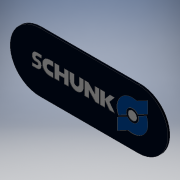
# Autodesk Inventor part: SCHUNK-9905502 Typenschild 9x24x0.3
Saved by Autodesk Inventor 2019 (Build 230136000, 136)
## iProperties
Created: 2022-08-29
Part Number: SCHUNK-9905502 Typenschild 9x24x0.3
Material: Generic
Catalog Web Link: www.cadenas.de
Description: Typenschild-SCHUNK-Typenschild
Vendor: SCHUNK
Document SubType Name: Modeling
Designer: psAdmin
Manufacturer: SCHUNK
Mass: 0.0577878 g
Surface Area: 4.19568 cm^2
Volume: 0.0577878 cm^3
Density: 1 g/cm^3
Appearance: PSOLRGB-175-175-175
Category: PARTsolutions
Company: SCHUNK
Title: SCHUNK-9905502 Typenschild 9x24x0.3
Author: Cadenas PARTsolutions
Comments: SCHUNK-Typenschild
PSOL_IDENT_0: {$CADENAS_DATA/23d-libs/schunk/normteile/typenschilder.prj},215 {VTYP=3D},{NB=SCHUNK-9905502 Typensc
PSOL_IDENT_1: hild 9x24x0.3},{LINA=SCHUNK-9905502 Typenschild 9x24x0.3},{NN=Typenschild},{DATE=31.03.2022 08:21:34
PSOL_IDENT_2: },{GEOMDATE=22.02.2022 09:18:32},{VERSION=},{LINEID=40},{WBVAR=},{WBNUMERIC=}  {NB=SCHUNK-9905502 Ty
PSOL_IDENT_3: penschild 9x24x0.3},{LINA=SCHUNK-9905502 Typenschild 9x24x0.3},{KT=DUMMY},{IDNR=9905502},{TYP=9x24x0
PSOL_IDENT_4: .3},{B=9.000},{L=24.000},{H=0.300},{SF=3.000},{SFL=2.800},{SFS=0.185},{SFBS=2.350},{VBS=-0.320},{VBC=
PSOL_IDENT_5: -0.400},{VBU=0.410},{VL=6.600},{VS=-36.900},{TYP1=4.000},{PARTSERVER=1.000}
NB: SCHUNK-9905502 Typenschild 9x24x0.3
NN: Typenschild
NT: SCHUNK-Typenschild
NBSYN: SCHUNK-$IDNR. Typenschild $TYP.
LINA: SCHUNK-9905502 Typenschild 9x24x0.3
CATALOG: SCHUNK
IDNR: 9905502
TYP: 9x24x0.3
B: 9
L: 24
H: 0.3
SF: 3
SFL: 2.8
SFS: 0.185
SFBS: 2.35
VBS: -0.32
VBC: -0.4
VBU: 0.41
VL: 6.6
VS: -36.9
TYP1: 4
PARTSERVER: 1
SUPPLIER: SCHUNK
ARTICLENO: SCHUNK-9905502 Typenschild 9x24x0.3
BOMINFO: SCHUNK-9905502 Typenschild 9x24x0.3
CREATOR: CADENAS GmbH
Autodesk Inventor part; units mm, degrees
sketch "Sketch_1" plane through (0, 0, 0) normal (0, 0, 1) x (1, 0, 0)
  arc A0 (-12, 0) -> (-7.5, -4.5) centre (-7.5, 0) ccw
  line L0 (-7.5, -4.5) -> (7.5, -4.5)
  arc A1 (7.5, -4.5) -> (12, 0) centre (7.5, 0) ccw
  arc A2 (12, 0) -> (7.5, 4.5) centre (7.5, 0) ccw
  line L1 (7.5, 4.5) -> (-7.5, 4.5)
  arc A3 (-7.5, 4.5) -> (-12, 0) centre (-7.5, 0) ccw
  constraints: 8 point on circle, 4 centre point, 4 end point
extrude "Extrusion1" add sketch "Sketch_1" along normal blind 0.3
sketch "Sketch_13" plane through (0, 0, 0.3) normal (0, 0, 1) x (1, 0, 0)
  line L0 (-5.2261, 1.0265) -> (-5.2261, -1.027)
  line L1 (-5.2261, -1.027) -> (-4.5423, -1.027)
  line L2 (-4.5423, -1.027) -> (-4.5423, -0.2502)
  line L3 (-4.5423, -0.2502) -> (-3.7899, -0.2502)
  line L4 (-3.7899, -0.2502) -> (-3.7899, -1.027)
  line L5 (-3.7899, -1.027) -> (-3.106, -1.027)
  line L6 (-3.106, -1.027) -> (-3.106, 1.0265)
  line L7 (-3.106, 1.0265) -> (-3.7899, 1.0265)
  line L8 (-3.7899, 1.0265) -> (-3.7899, 0.2798)
  line L9 (-3.7899, 0.2798) -> (-4.5423, 0.2798)
  line L10 (-4.5423, 0.2798) -> (-4.5423, 1.0265)
  line L11 (-4.5423, 1.0265) -> (-5.2261, 1.0265)
  constraints: 24 end point
extrude "Extrusion2" cut sketch "Sketch_13" against normal blind 0.05
sketch "Sketch_15" plane through (0, 0, 0.3) normal (0, 0, 1) x (1, 0, 0)
  line L0 (-0.689, 1.0265) -> (-0.689, -1.027)
  line L1 (-0.689, -1.027) -> (-0.0337, -1.027)
  line L2 (-0.0337, -1.027) -> (-0.0337, 0.0269)
  line L3 (-0.0337, 0.0269) -> (0.9535, -1.027)
  line L4 (0.9535, -1.027) -> (1.537, -1.027)
  line L5 (1.537, -1.027) -> (1.537, 1.0265)
  line L6 (1.537, 1.0265) -> (0.8819, 1.0265)
  line L7 (0.8819, 1.0265) -> (0.8819, -0.0273)
  line L8 (0.8819, -0.0273) -> (-0.1051, 1.0265)
  line L9 (-0.1051, 1.0265) -> (-0.689, 1.0265)
  constraints: 20 end point
extrude "Extrusion3" cut sketch "Sketch_15" against normal blind 0.05
sketch "Sketch_16" plane through (0, 0, 0.3) normal (0, 0, 1) x (1, 0, 0)
  line L0 (1.7129, 1.0265) -> (1.7129, -1.027)
  line L1 (1.7129, -1.027) -> (2.3967, -1.027)
  line L2 (2.3967, -1.027) -> (2.3967, -0.0588)
  line L3 (2.3967, -0.0588) -> (3.1093, -1.027)
  line L4 (3.1093, -1.027) -> (3.9246, -1.027)
  line L5 (3.9246, -1.027) -> (3.1004, 0.0719)
  line L6 (3.1004, 0.0719) -> (3.8959, 1.0265)
  line L7 (3.8959, 1.0265) -> (3.1777, 1.0265)
  line L8 (3.1777, 1.0265) -> (2.3967, 0.0961)
  line L9 (2.3967, 0.0961) -> (2.3967, 1.0265)
  line L10 (2.3967, 1.0265) -> (1.7129, 1.0265)
  constraints: 22 end point
extrude "Extrusion4" cut sketch "Sketch_16" against normal blind 0.05
sketch "Sketch_5" plane through (0, 0, 0.3) normal (0, 0, 1) x (1, 0, 0)
  arc A0 (-8.6625, 0.2585) -> (-8.1925, -0.2115) centre (-8.1925, 0.2585) ccw
  line L0 (-8.1925, -0.2115) -> (-7.9457, -0.2115)
  arc A1 (-7.9457, -0.611) -> (-7.9457, -0.2115) centre (-7.9457, -0.4113) ccw
  line L1 (-7.9457, -0.611) -> (-8.6625, -0.611)
  line L2 (-8.6625, -0.611) -> (-8.6625, -1.0575)
  line L3 (-8.6625, -1.0575) -> (-7.9105, -1.0575)
  arc A2 (-7.9105, -1.0575) -> (-7.2525, -0.3995) centre (-7.9105, -0.3995) ccw
  line L4 (-7.2525, -0.3995) -> (-7.2525, -0.2585)
  arc A3 (-7.2525, -0.2585) -> (-7.7225, 0.2115) centre (-7.7225, -0.2585) ccw
  line L5 (-7.7225, 0.2115) -> (-7.9457, 0.2115)
  arc A4 (-7.9457, 0.611) -> (-7.9457, 0.2115) centre (-7.9395, 0.4113) ccw
  line L6 (-7.9457, 0.611) -> (-7.2525, 0.611)
  line L7 (-7.2525, 0.611) -> (-7.2525, 1.0575)
  line L8 (-7.2525, 1.0575) -> (-8.0045, 1.0575)
  arc A5 (-8.0045, 1.0575) -> (-8.6625, 0.3995) centre (-8.0045, 0.3995) ccw
  line L9 (-8.6625, 0.3995) -> (-8.6625, 0.2585)
  constraints: 20 end point, 12 point on circle, 6 centre point
extrude "Extrusion5" cut sketch "Sketch_5" against normal blind 0.05
sketch "Sketch_6" plane through (0, 0, 0.3) normal (0, 0, 1) x (1, 0, 0)
  arc A0 (-6.04, 1.0693) -> (-6.04, -1.0693) centre (-6.04, 0) ccw
  line L0 (-6.04, -1.0693) -> (-5.429, -1.0693)
  line L1 (-5.429, -1.0693) -> (-5.429, -0.3995)
  line L2 (-5.429, -0.3995) -> (-6.04, -0.3995)
  arc A1 (-6.04, 0.3995) -> (-6.04, -0.3995) centre (-6.04, 0) ccw
  line L3 (-6.04, 0.3995) -> (-5.429, 0.3995)
  line L4 (-5.429, 0.3995) -> (-5.429, 1.0693)
  line L5 (-5.429, 1.0693) -> (-6.04, 1.0693)
  constraints: 12 end point, 4 point on circle, 2 centre point
extrude "Extrusion6" cut sketch "Sketch_6" against normal blind 0.05
sketch "Sketch_7" plane through (0, 0, 0.3) normal (0, 0, 1) x (1, 0, 0)
  line L0 (-2.948, 1.034) -> (-2.948, 0)
  arc A0 (-2.948, 0) -> (-0.833, 0) centre (-1.8905, 0) ccw
  line L1 (-0.833, 0) -> (-0.833, 1.034)
  line L2 (-0.833, 1.034) -> (-1.5145, 1.034)
  line L3 (-1.5145, 1.034) -> (-1.5145, 0)
  arc A1 (-2.2665, 0) -> (-1.5145, 0) centre (-1.8905, 0) ccw
  line L4 (-2.2665, 0) -> (-2.2665, 1.034)
  line L5 (-2.2665, 1.034) -> (-2.948, 1.034)
  constraints: 12 end point, 4 point on circle, 2 centre point
extrude "Extrusion7" cut sketch "Sketch_7" against normal blind 0.05
sketch "Sketch8" plane through (0, 0, 0.3) normal (0, 0, 1) x (1, 0, 0)
  point P0 (6.6, 0)
hole "Hole1" at (6.6, 0, 0.3) direction (0, 0, -1) diameter 1.344 depth 0.05
sketch "Sketch_3" plane through (0, 0, 0.3) normal (0, 0, 1) x (1, 0, 0)
  arc A0 (7.2909, 2.2698) -> (4.4594, -1.0234) centre (6.6, 0) ccw
  line L0 (4.4594, -1.0234) -> (5.7362, -0.352)
  arc A1 (7.3714, 0.5243) -> (5.7362, -0.352) centre (6.6, 0) ccw
  line L1 (7.3714, 0.5243) -> (8.9464, 1.3615)
  line L2 (8.9464, 1.3615) -> (8.9464, 3.1479)
  line L3 (8.9464, 3.1479) -> (7.2909, 2.2698)
  constraints: 8 end point, 4 point on circle, 2 centre point
extrude "Extrusion8" cut sketch "Sketch_3" against normal blind 0.05
sketch "Sketch_4" plane through (0, 0, 0.3) normal (0, 0, 1) x (1, 0, 0)
  line L0 (4.262, -1.3559) -> (4.262, -3.1423)
  line L1 (4.262, -3.1423) -> (5.9182, -2.2715)
  arc A0 (5.9182, -2.2715) -> (8.7347, 1.0332) centre (6.6, 0) ccw
  line L2 (8.7347, 1.0332) -> (7.4617, 0.3479)
  arc A1 (5.8342, -0.5264) -> (7.4617, 0.3479) centre (6.6, 0) ccw
  line L3 (5.8342, -0.5264) -> (4.262, -1.3559)
  constraints: 8 end point, 4 point on circle, 2 centre point
extrude "Extrusion9" cut sketch "Sketch_4" against normal blind 0.05
ref_plane "aluschild_XY" through (0, 0, 0) normal (0, 0, 1) x (1, 0, 0)
ref_plane "aluschild_YZ" through (0, 0, 0) normal (1, 0, 0) x (0, 1, 0)
ref_plane "aluschild_ZX" through (0, 0, 0) normal (0, 1, 0) x (0, 0, 1)
body "Solid1"
